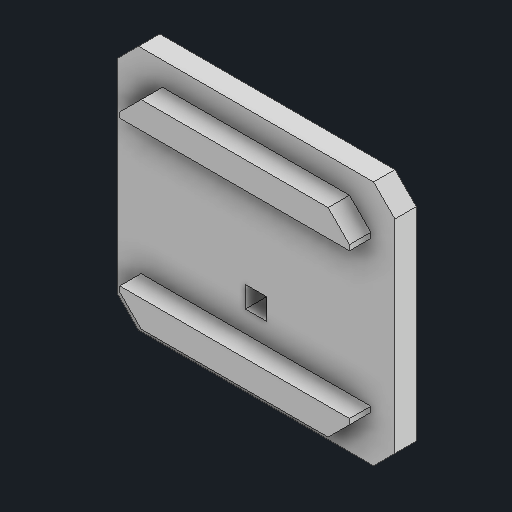
# Autodesk Inventor part: TampaEletronica
Saved by Autodesk Inventor 2027 (Build 310192000, 192)
## iProperties
Created: 2026-07-11
Part Number: TampaEletronica
Material: Genérico
Document SubType Name: Modeling
Designer: marcu
Mass: 1.371 g
Surface Area: 15.5725 cm^2
Volume: 1.371 cm^3
Density: 1 g/cm^3
Appearance: Padrão
Author: marcu
Autodesk Inventor part; units mm, degrees
ref_plane "YZ Plane" through (0, 0, 0) normal (1, 0, 0) x (0, 1, 0)
ref_plane "XZ Plane" through (0, 0, 0) normal (0, 1, 0) x (-1, 0, 0)
ref_plane "XY Plane" through (0, 0, 0) normal (0, 0, 1) x (1, 0, 0)
sketch "Esboço1" plane through (0, 0, 0) normal (0, 0, 1) x (1, 0, 0)
  line L0 (-13, 11.5) -> (13, 11.5)
  line L1 (13, 11.5) -> (13, -11.5)
  line L2 (13, -11.5) -> (-13, -11.5)
  line L3 (-13, -11.5) -> (-13, 11.5)
  line L4 (-13, 11.5) -> (13, -11.5) construction
  line L5 (13, 11.5) -> (-13, -11.5) construction
  point P0 (0, 0)
  dimension "d0" = 26
  dimension "d1" = 23
  constraints: 12 end point, 2 midpoint, 2 parallel, 1 horizontal, 1 perpendicular
  measures "d0" distance of L1.end L2.end
  measures "d1" distance of L0.end L1.end
extrude "Extrusão1" add sketch "Esboço1" along normal blind 2
chamfer "Chanfro1" distance 2 angle 45 4 edges at (-13, 11.5, 1) (-13, -11.5, 1) (13, 11.5, 1) (13, -11.5, 1)
sketch "Esboço2" plane through (0, 0, 2) normal (0, 0, 1) x (1, 0, 0)
  line L0 (-10.75, 6.8) -> (10.75, 6.8)
  line L1 (10.75, 6.8) -> (10.75, 9.3)
  line L2 (10.75, 9.3) -> (-10.75, 9.3)
  line L3 (-10.75, 9.3) -> (-10.75, 6.8)
  line L4 (-10.75, 6.8) -> (10.75, 9.3) construction
  line L5 (10.75, 6.8) -> (-10.75, 9.3) construction
  line L6 (11, 11.5) -> (-11, 11.5) projected
  line L7 (-13, 9.5) -> (-13, -9.5) projected
  line L8 (0, 0) -> (3.5372, 0) construction
  line L9 (-10.75, -6.8) -> (10.75, -6.8)
  line L10 (10.75, -6.8) -> (10.75, -9.3)
  line L11 (10.75, -9.3) -> (-10.75, -9.3)
  line L12 (-10.75, -9.3) -> (-10.75, -6.8)
  line L13 (-10.75, -6.8) -> (10.75, -9.3) construction
  line L14 (10.75, -6.8) -> (-10.75, -9.3) construction
  point P0 (0, 8.05)
  point P1 (0, -8.05)
  dimension "d7" = 21.5
  dimension "d8" = 2.5
  dimension "d9" = 2.2
  dimension "d10" = 2.25
  constraints: 26 end point, 5 symmetric about line, 2 horizontal, 2 midpoint, 2 parallel, 1 perpendicular
  measures "d7" distance of L1.end L2.end
  measures "d8" distance of L1.end L0.end
  measures "d9" distance between parallel lines of L6 L2
  measures "d10" distance between parallel lines of L3 L7
extrude "Extrusão2" add sketch "Esboço2" along normal blind 2
chamfer "Chanfro2" distance 2 angle 45 4 edges at (-10.75, 9.3, 3) (10.75, 9.3, 3) (10.75, -9.3, 3) (-10.75, -9.3, 3)
sketch "Esboço3" plane through (0, 0, 2) normal (0, 0, 1) x (1, 0, 0)
  line L0 (-1, -2.8) -> (1, -2.8)
  line L1 (1, -2.8) -> (1, -4.8)
  line L2 (1, -4.8) -> (-1, -4.8)
  line L3 (-1, -4.8) -> (-1, -2.8)
  line L4 (-1, -2.8) -> (1, -4.8) construction
  line L5 (1, -2.8) -> (-1, -4.8) construction
  line L6 (-10.75, -6.8) -> (10.75, -6.8) projected
  line L7 (13, -9.5) -> (13, 9.5) projected
  point P0 (0, 0)
  point P1 (0, -3.8)
  dimension "d16" = 2
  dimension "d17" = 2
  dimension "d18" = 2
  dimension "d19" = 12
  constraints: 12 end point, 2 midpoint, 2 parallel, 1 horizontal, 1 perpendicular
  measures "d16" distance of L1.end L2.end
  measures "d17" distance of L0.end L1.end
  measures "d18" distance between parallel lines of L6 L2
  measures "d19" distance between parallel lines of L7 L1
extrude "Extrusão3" cut sketch "Esboço3" against normal blind 10
